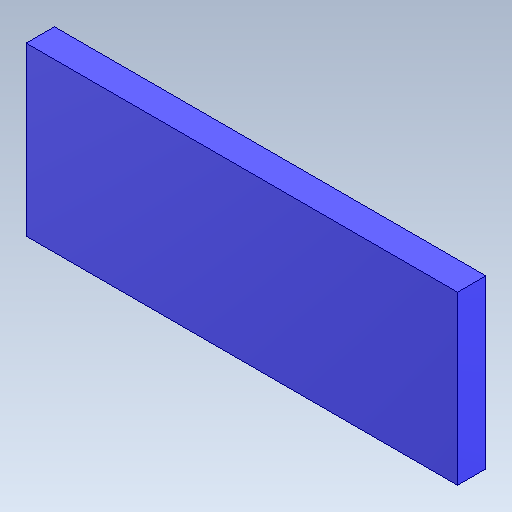
# Autodesk Inventor part: 22-27-2061-06
Saved by Autodesk Inventor 2020 (Build 240168000, 168)
## iProperties
Created: 2019-08-29
Part Number: 22-27-2061-06
Material: Generic
Document SubType Name: Modeling
Designer: psrob
Density: 1 g/cm^3
Appearance: 6410-06, 22-27-2061-06
Author: psrob
Autodesk Inventor part; units mm, degrees
ref_plane "YZ Plane" through (0, 0, 0) normal (1, 0, 0) x (0, 1, 0)
ref_plane "XZ Plane" through (0, 0, 0) normal (0, 1, 0) x (-1, 0, 0)
ref_plane "XY Plane" through (0, 0, 0) normal (0, 0, 1) x (1, 0, 0)
sketch "6410-06, 22-27-2061-06_32" plane through (0, 0, 0) normal (0, 0, 1) x (1, 0, 0)
  line L0 (-7.62, 2.9845) -> (7.62, 2.9845)
  line L1 (7.62, 2.9845) -> (7.62, -2.921)
  line L2 (7.62, -2.921) -> (-7.62, -2.921)
  line L3 (-7.62, -2.921) -> (-7.62, 2.9845)
  constraints: 8 end point
extrude "Extrusion1" add sketch "6410-06, 22-27-2061-06_32" along normal blind 1
body "Solid1"
